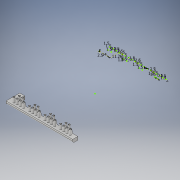
# Autodesk Inventor part: 24WellPlateConnectorV2
Saved by Autodesk Inventor 2019 (Build 230136000, 136)
## iProperties
Created: 2019-12-12
Part Number: 24WellPlateConnectorV2
Material: Generic
Document SubType Name: Modeling
Designer: Sergio
Density: 1 g/cm^3
Appearance: Default
Author: Sergio
Autodesk Inventor part; units mm, degrees
ref_plane "YZ Plane" through (0, 0, 0) normal (1, 0, 0) x (0, 1, 0)
ref_plane "XZ Plane" through (0, 0, 0) normal (0, 1, 0) x (-1, 0, 0)
ref_plane "XY Plane" through (0, 0, 0) normal (0, 0, 1) x (1, 0, 0)
sketch "Sketch1" plane through (0, 0, 0) normal (0, 1, 0) x (-1, 0, 0)
  circle A0 centre (39.0419, -55.5191) radius 0.75 construction
  circle A1 centre (41.3055, -60.0191) radius 0.75 construction
  circle A2 centre (37.3055, -60.0191) radius 0.75 construction
  circle A3 centre (35.0419, -55.5191) radius 0.75 construction
  circle A4 centre (33.3055, -60.0191) radius 0.75 construction
  circle A5 centre (29.3055, -60.0191) radius 0.75 construction
  line L0 (33.0555, -60.0191) -> (33.5555, -60.0191) construction
  line L1 (37.0555, -60.0191) -> (37.5555, -60.0191) construction
  circle A6 centre (39.0419, -55.5191) radius 0.75 construction
  circle A7 centre (41.3055, -60.0191) radius 0.75 construction
  circle A8 centre (37.3055, -60.0191) radius 0.75 construction
  circle A9 centre (35.0419, -55.5191) radius 0.75 construction
  circle A10 centre (29.3055, -60.0191) radius 0.75 construction
  circle A11 centre (33.3055, -60.0191) radius 0.75 construction
  circle A12 centre (9.8055, -60.0191) radius 0.75 construction
  circle A13 centre (13.8055, -60.0191) radius 0.75 construction
  line L2 (13.5555, -60.0191) -> (14.0555, -60.0191) construction
  circle A14 centre (15.5419, -55.5191) radius 0.75 construction
  circle A15 centre (17.8055, -60.0191) radius 0.75 construction
  circle A16 centre (19.5419, -55.5191) radius 0.75 construction
  circle A17 centre (21.8055, -60.0191) radius 0.75 construction
  circle A18 centre (-9.6945, -60.0191) radius 0.75 construction
  circle A19 centre (-5.6945, -60.0191) radius 0.75 construction
  circle A20 centre (-3.9581, -55.5191) radius 0.75 construction
  circle A21 centre (-1.6945, -60.0191) radius 0.75 construction
  circle A22 centre (0.0419, -55.5191) radius 0.75 construction
  circle A23 centre (2.3055, -60.0191) radius 0.75 construction
  circle A24 centre (-29.1945, -60.0191) radius 0.75 construction
  circle A25 centre (-25.1945, -60.0191) radius 0.75 construction
  circle A26 centre (-23.4581, -55.5191) radius 0.75 construction
  line L3 (-21.4445, -60.0191) -> (-20.9445, -60.0191) construction
  circle A27 centre (-21.1945, -60.0191) radius 0.75 construction
  circle A28 centre (-19.4581, -55.5191) radius 0.75 construction
  circle A29 centre (-17.1945, -60.0191) radius 0.75 construction
  circle A30 centre (29.3055, -60.0191) radius 0.75 construction
  circle A31 centre (21.8055, -60.0191) radius 0.75 construction
  circle A32 centre (2.3055, -60.0191) radius 0.75 construction
  circle A33 centre (9.8055, -60.0191) radius 0.75 construction
  circle A34 centre (-17.1945, -60.0191) radius 0.75 construction
  circle A35 centre (-9.6945, -60.0191) radius 0.75 construction
  line L4 (21.8055, -60.0191) -> (29.3055, -60.0191) construction
  line L5 (2.3055, -60.0191) -> (9.8055, -60.0191) construction
  arc A36 (-17.4445, -59.312) -> (-16.9445, -59.312) centre (-17.1945, -60.0191) ccw construction
  line L6 (-17.1945, -60.0191) -> (-9.6945, -60.0191) construction
  circle A37 centre (25.5555, -60.0191) radius 1.25 construction
  circle A38 centre (6.0555, -60.0191) radius 1.25 construction
  circle A39 centre (-13.4445, -60.0191) radius 1.25 construction
  line L7 (29.3055, -60.0191) -> (29.3055, -48.7591) construction
  line L8 (29.3055, -48.7591) -> (43.3055, -48.7591) construction
  circle A40 centre (43.3055, -48.7591) radius 1.25 construction
  point P0 (-21.1945, -55.9676)
  point P1 (0, 0)
  dimension "d6" = 0.5
  dimension "d8" = 0.5
  dimension "d18" = 1.5
  dimension "d19" = 1.5
  dimension "d21" = 1.5
  dimension "d22" = 1.5
  dimension "d29" = 0.5
  dimension "d40" = 1.5
  dimension "d41" = 1.5
  dimension "d42" = 1.5
  dimension "d43" = 1.5
  dimension "d44" = 1.5
  dimension "d45" = 1.5
  dimension "d63" = 1.5
  dimension "d64" = 1.5
  dimension "d65" = 1.5
  dimension "d68" = 1.5
  dimension "d77" = 0.5
  dimension "d86" = 1.5
  dimension "d87" = 1.5
  dimension "d88" = 1.5
  dimension "d89" = 1.5
  dimension "d90" = 1.5
  dimension "d91" = 1.5
  dimension "d97" = 2.5
  dimension "d98" = 2.5
  dimension "d99" = 2.5
  dimension "d141" = 11.26
  dimension "d142" = 14
  dimension "d143" = 2.5
  constraints: 41 centre point, 18 end point, 7 coincident, 3 horizontal, 2 point on circle, 1 midpoint, 1 perpendicular, 1 vertical
  measures "d6" distance of L0.end L0.start
  measures "d8" distance of L1.end L1.start
  measures "d18" diameter of A7
  measures "d19" diameter of A8
  measures "d21" diameter of A10
  measures "d22" diameter of A11
  measures "d29" distance of L2.end L2.start
  measures "d40" diameter of A16
  measures "d41" diameter of A17
  measures "d42" diameter of A15
  measures "d43" diameter of A14
  measures "d44" diameter of A12
  measures "d45" diameter of A13
  measures "d63" diameter of A22
  measures "d64" diameter of A23
  measures "d65" diameter of A21
  measures "d68" diameter of A19
  measures "d77" distance of L3.end L3.start
  measures "d86" diameter of A28
  measures "d87" diameter of A29
  measures "d88" diameter of A27
  measures "d89" diameter of A26
  measures "d90" diameter of A24
  measures "d91" diameter of A25
  measures "d97" diameter of A37
  measures "d98" diameter of A38
  measures "d99" diameter of A39
  measures "d141" distance of L4.end L7.end
  measures "d142" distance of L7.end L8.end
  measures "d143" diameter of A40
sketch "Sketch2" plane through (0, 0, 0) normal (0, 1, 0) x (-1, 0, 0)
  circle A0 centre (-29.1945, -60.0191) radius 0.75 construction
  circle A1 centre (-23.4581, -55.5191) radius 0.75 construction
  circle A2 centre (-25.1945, -60.0191) radius 0.75 construction
  circle A3 centre (-21.1945, -60.0191) radius 0.75 construction
  circle A4 centre (-19.4581, -55.5191) radius 0.75 construction
  circle A5 centre (-17.1945, -60.0191) radius 0.75 construction
  circle A6 centre (-9.6945, -60.0191) radius 0.75 construction
  circle A7 centre (9.8055, -60.0191) radius 0.75 construction
  circle A8 centre (29.3055, -60.0191) radius 0.75 construction
  circle A9 centre (-29.1945, -60.0191) radius 0.95
  circle A10 centre (-25.1945, -60.0191) radius 0.95
  circle A11 centre (-23.4581, -55.5191) radius 0.95
  circle A12 centre (-19.4581, -55.5191) radius 0.95
  circle A13 centre (-21.1945, -60.0191) radius 1.1
  circle A14 centre (-17.1945, -60.0191) radius 0.95
  circle A15 centre (6.0555, -60.0191) radius 1.25 construction
  circle A16 centre (25.5555, -60.0191) radius 1.25 construction
  circle A17 centre (-9.6945, -60.0191) radius 0.95
  circle A18 centre (-5.6945, -60.0191) radius 0.95
  circle A19 centre (-3.9581, -55.5191) radius 0.95
  circle A20 centre (0.0419, -55.5191) radius 0.95
  circle A21 centre (-1.6945, -60.0191) radius 0.95
  circle A22 centre (2.3055, -60.0191) radius 0.95
  circle A23 centre (9.8055, -60.0191) radius 0.95
  circle A24 centre (13.8055, -60.0191) radius 0.95
  circle A25 centre (15.5419, -55.5191) radius 0.95
  circle A26 centre (19.5419, -55.5191) radius 0.95
  circle A27 centre (17.8055, -60.0191) radius 0.95
  circle A28 centre (21.8055, -60.0191) radius 0.95
  circle A29 centre (29.3055, -60.0191) radius 0.95
  circle A30 centre (33.3055, -60.0191) radius 0.95
  circle A31 centre (35.0419, -55.5191) radius 0.95
  circle A32 centre (39.0419, -55.5191) radius 0.95
  circle A33 centre (37.3055, -60.0191) radius 0.95
  circle A34 centre (41.3055, -60.0191) radius 0.95
  line L0 (6.0555, -56.0191) -> (6.0555, -42.498) construction
  line L1 (-29.1945, -60.0191) -> (-29.1945, -63.4191) construction
  line L2 (41.3055, -60.0191) -> (41.3055, -63.4191) construction
  line L3 (-29.1945, -63.4191) -> (41.3055, -63.4191) construction
  circle A35 centre (43.3055, -48.7591) radius 1.25 construction
  point P0 (0, 0)
  dimension "d110" = 1.9
  dimension "d111" = 1.9
  dimension "d112" = 1.9
  dimension "d113" = 1.9
  dimension "d114" = 2.2
  dimension "d115" = 1.9
  dimension "d121" = 1.9
  dimension "d122" = 1.9
  dimension "d123" = 1.9
  dimension "d124" = 1.9
  dimension "d125" = 1.9
  dimension "d126" = 1.9
  dimension "d127" = 1.9
  dimension "d128" = 1.9
  dimension "d129" = 1.9
  dimension "d130" = 1.9
  dimension "d131" = 1.9
  dimension "d132" = 1.9
  dimension "d133" = 1.9
  dimension "d134" = 1.9
  dimension "d135" = 1.9
  dimension "d136" = 1.9
  dimension "d137" = 1.9
  dimension "d138" = 1.9
  dimension "d139" = 3.4
  dimension "d140" = 3.4
  constraints: 24 centre point, 8 end point, 6 coincident, 3 vertical, 1 horizontal
  measures "d110" diameter of A9
  measures "d111" diameter of A10
  measures "d112" diameter of A11
  measures "d113" diameter of A12
  measures "d114" diameter of A13
  measures "d115" diameter of A14
  measures "d121" diameter of A17
  measures "d122" diameter of A18
  measures "d123" diameter of A19
  measures "d124" diameter of A20
  measures "d125" diameter of A21
  measures "d126" diameter of A22
  measures "d127" diameter of A23
  measures "d128" diameter of A24
  measures "d129" diameter of A25
  measures "d130" diameter of A26
  measures "d131" diameter of A27
  measures "d132" diameter of A28
  measures "d133" diameter of A29
  measures "d134" diameter of A30
  measures "d135" diameter of A31
  measures "d136" diameter of A32
  measures "d137" diameter of A33
  measures "d138" diameter of A34
  measures "d139" distance of L1.start L1.end
  measures "d140" distance of L2.start L2.end
sketch "Sketch4" plane through (0, 0, 0) normal (0, 1, 0) x (-1, 0, 0)
  circle A0 centre (35.0419, -55.5191) radius 0.95 projected
  circle A1 centre (39.0419, -55.5191) radius 0.95 projected
  circle A2 centre (41.3055, -60.0191) radius 0.95 projected
  circle A3 centre (43.3055, -48.7591) radius 1.25 projected
  circle A4 centre (33.3055, -60.0191) radius 0.95 projected
  circle A5 centre (29.3055, -60.0191) radius 0.95 projected
  circle A6 centre (25.5555, -60.0191) radius 1.25 construction
  circle A7 centre (25.5555, -60.0191) radius 1.25 projected
  line L0 (41.3055, -60.0191) -> (45.3055, -60.0191) construction
  line L1 (43.3055, -48.7591) -> (41.3055, -48.7591) construction
  line L2 (43.3055, -48.7591) -> (43.3055, -46.2591) construction
  line L3 (39.0419, -55.5191) -> (39.0419, -52.5191) construction
  line L4 (35.0419, -55.5191) -> (35.0419, -52.5191) construction
  line L5 (29.3055, -60.0191) -> (29.3055, -57.0191) construction
  circle A8 centre (9.8055, -60.0191) radius 0.95 projected
  circle A9 centre (-9.6945, -60.0191) radius 0.95 projected
  circle A10 centre (-29.1945, -60.0191) radius 0.95 projected
  line L6 (-17.1945, -60.0191) -> (-13.1945, -60.0191) construction
  line L7 (-19.4581, -55.5191) -> (-19.4581, -52.5191) construction
  line L8 (-23.4581, -55.5191) -> (-23.4581, -52.5191) construction
  line L9 (-29.1945, -60.0191) -> (-29.1945, -57.0191) construction
  line L10 (2.3055, -60.0191) -> (6.3055, -60.0191) construction
  line L11 (0.0419, -55.5191) -> (0.0419, -52.5191) construction
  line L12 (-3.9581, -55.5191) -> (-3.9581, -52.5191) construction
  line L13 (-9.6945, -60.0191) -> (-9.6945, -57.0191) construction
  line L14 (21.8055, -60.0191) -> (25.8055, -60.0191) construction
  line L15 (19.5419, -55.5191) -> (19.5419, -52.5191) construction
  line L16 (15.5419, -55.5191) -> (15.5419, -52.5191) construction
  line L17 (9.8055, -60.0191) -> (9.8055, -57.0191) construction
  line L18 (39.0419, -52.5191) -> (41.3055, -48.7591)
  line L19 (41.3055, -48.7591) -> (41.3055, -46.2591)
  line L20 (41.3055, -46.2591) -> (47.8055, -46.2591)
  line L21 (21.8055, -60.0191) -> (21.8055, -57.0191) construction
  line L22 (2.3055, -60.0191) -> (2.3055, -57.0191) construction
  line L23 (-17.1945, -60.0191) -> (-17.1945, -57.0191) construction
  line L24 (19.5419, -52.5191) -> (15.5419, -52.5191)
  line L25 (9.8055, -57.0191) -> (15.5419, -52.5191)
  line L26 (0.0419, -52.5191) -> (-3.9581, -52.5191)
  line L27 (-9.6945, -57.0191) -> (-3.9581, -52.5191)
  line L28 (-23.4581, -52.5191) -> (-19.4581, -52.5191)
  line L29 (-29.1945, -57.0191) -> (-23.4581, -52.5191)
  line L30 (-29.1945, -57.0191) -> (-35.6945, -57.0191)
  line L31 (-29.1945, -63.4191) -> (41.3055, -63.4191) construction
  line L32 (-35.6945, -57.0191) -> (-35.6945, -63.4191)
  line L33 (-35.6945, -63.4191) -> (47.8055, -63.4191)
  line L34 (47.8055, -63.4191) -> (47.8055, -46.2591)
  line L35 (29.3055, -57.0191) -> (24.3055, -57.0191)
  line L36 (24.3055, -57.0191) -> (19.5419, -52.5191)
  line L37 (9.8055, -57.0191) -> (4.8055, -57.0191)
  line L38 (4.8055, -57.0191) -> (0.0419, -52.5191)
  line L39 (-9.6945, -57.0191) -> (-14.6945, -57.0191)
  line L40 (-14.6945, -57.0191) -> (-19.4581, -52.5191)
  line L41 (29.3055, -57.0191) -> (36.3055, -57.0191) construction
  line L42 (39.0419, -52.5191) -> (35.0419, -52.5191)
  line L43 (35.0419, -52.5191) -> (29.3055, -57.0191)
  line L44 (41.3055, -60.0191) -> (44.5555, -60.0191)
  point P0 (0, 0)
  dimension "d145" = 4
  dimension "d146" = 2
  dimension "d147" = 2.5
  dimension "d150" = 3
  dimension "d151" = 4
  dimension "d152" = 3
  dimension "d153" = 3
  dimension "d154" = 3
  dimension "d155" = 4
  dimension "d156" = 3
  dimension "d157" = 3
  dimension "d158" = 3
  dimension "d159" = 4
  dimension "d160" = 3
  dimension "d161" = 3
  dimension "d162" = 3
  dimension "d163" = 6.5
  dimension "d164" = 3
  dimension "d165" = 3
  dimension "d166" = 3
  dimension "d167" = 6.5
  dimension "d168" = 5
  dimension "d169" = 5
  dimension "d170" = 5
  constraints: 88 end point, 19 vertical, 12 horizontal, 1 parallel, 1 perpendicular, 1 point on line
  measures "d145" distance of L0.start L0.end
  measures "d146" distance of L1.start L1.end
  measures "d147" distance of L1.start L2.end
  measures "d150" distance of L5.start L5.end
  measures "d151" distance of L6.start L6.end
  measures "d152" distance of L7.start L7.end
  measures "d153" distance of L8.start L8.end
  measures "d154" distance of L9.start L9.end
  measures "d155" distance of L10.start L10.end
  measures "d156" distance of L11.start L11.end
  measures "d157" distance of L12.start L12.end
  measures "d158" distance of L13.start L13.end
  measures "d159" distance of L14.start L14.end
  measures "d160" distance of L15.start L15.end
  measures "d161" distance of L16.start L16.end
  measures "d162" distance of L17.start L17.end
  measures "d163" distance of L19.end L20.end
  measures "d164" distance of L14.start L21.end
  measures "d165" distance of L10.start L22.end
  measures "d166" distance of L6.start L23.end
  measures "d167" distance of L9.end L30.end
  measures "d168" distance of L5.end L35.end
  measures "d169" distance of L17.end L37.end
  measures "d170" distance of L13.end L39.end
extrude "Extrusion1" add sketch "Sketch4" against normal blind 4 contours A0 | A1 | A2 | A3 | A4 | A5 | A7 | A8 | A9 | A10 | L18 L19 L20 L34 L33 L32 L30 L29 L28 L40 L39 L27 L26 L38 L37 L25 L24 L36 L35 L43 L42
sketch "Sketch5" plane through (0, 0, 0) normal (0, 1, 0) x (1, 0, 0)
  circle A0 centre (25.1945, 60.0191) radius 0.75 construction
  line L0 (25.1945, 60.0191) -> (26.4692, 60.0191) construction
  circle A1 centre (23.4581, 55.5191) radius 0.75 construction
  circle A2 centre (21.1945, 60.0191) radius 0.75 construction
  circle A3 centre (19.4581, 55.5191) radius 0.75 construction
  circle A4 centre (17.1945, 60.0191) radius 0.75 construction
  circle A5 centre (5.6945, 60.0191) radius 0.75 construction
  circle A6 centre (3.9581, 55.5191) radius 0.75 construction
  circle A7 centre (1.6945, 60.0191) radius 0.75 construction
  circle A8 centre (-0.0419, 55.5191) radius 0.75 construction
  circle A9 centre (-2.3055, 60.0191) radius 0.75 construction
  circle A10 centre (-9.8055, 60.0191) radius 0.75 construction
  circle A11 centre (-13.8055, 60.0191) radius 0.75 construction
  circle A12 centre (-15.5419, 55.5191) radius 0.75 construction
  circle A13 centre (-17.8055, 60.0191) radius 0.75 construction
  circle A14 centre (-35.0419, 55.5191) radius 0.75 construction
  circle A15 centre (-39.0419, 55.5191) radius 0.75 construction
  circle A16 centre (-41.3055, 60.0191) radius 0.75 construction
  circle A17 centre (-37.3055, 60.0191) radius 0.75 construction
  circle A18 centre (-19.5419, 55.5191) radius 0.75 construction
  circle A19 centre (-21.8055, 60.0191) radius 0.75 construction
  circle A20 centre (-29.3055, 60.0191) radius 0.75 construction
  circle A21 centre (-33.3055, 60.0191) radius 0.75 construction
  circle A22 centre (29.1945, 60.0191) radius 0.75 construction
  circle A23 centre (9.6945, 60.0191) radius 0.75 construction
  point P0 (0, 0)
  constraints: 24 coincident, 2 end point, 1 horizontal
fillet "Fillet1" radius 2 1 edges at (-6.0555, -4, -63.4191)
extrude "Extrusion6" add sketch "Sketch2" along normal blind 6 contours A13
sketch "Sketch13" plane through (21.1945, 6, -60.0191) normal (0, 1, 0) x (1, 0, 0)
  circle A0 centre (0, 0) radius 1.1 projected
  circle A1 centre (0, 0) radius 0.775
  point P0 (-21.1945, -60.0191)
  dimension "d210" = 1.55
  constraints: 1 centre point, 1 coincident
  measures "d210" diameter of A1
extrude "Extrusion7" cut sketch "Sketch13" against normal blind 3 contours A1
pattern_sketch "Sketch Driven Pattern4" of "Extrusion6", "Extrusion7" from (21.1945, 0, -60.0191) copies at (23.4581, 0, -55.5191) at (19.4581, 0, -55.5191) at (17.1945, 0, -60.0191) at (5.6945, 0, -60.0191) at (1.6945, 0, -60.0191) at (-2.3055, 0, -60.0191) at (-0.0419, 0, -55.5191) at (3.9581, 0, -55.5191) at (-9.8055, 0, -60.0191) at (-13.8055, 0, -60.0191) at (-15.5419, 0, -55.5191) at (-17.8055, 0, -60.0191) at (-19.5419, 0, -55.5191) at (-21.8055, 0, -60.0191) at (-29.3055, 0, -60.0191) at (-33.3055, 0, -60.0191) at (-35.0419, 0, -55.5191) at (-37.3055, 0, -60.0191) at (-39.0419, 0, -55.5191) at (-41.3055, 0, -60.0191) at (29.1945, 0, -60.0191) at (9.6945, 0, -60.0191) at (25.1945, 0, -60.0191)
mirror "Mirror7" about plane through (0, 0, 0) normal (0, 0, 1) remove original yes
body "Solid1"
